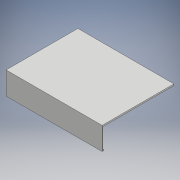
# Autodesk Inventor part: 包包分隔檔板
Saved by Autodesk Inventor 2017 (Build 210142000, 142)
## iProperties
Part Number: 包包分隔檔板
Material: 一般
Document SubType Name: Modeling
Designer: user
Density: 1 g/cm^3
Appearance: 預設
Author: user
Autodesk Inventor part; units mm, degrees
ref_plane "YZ Plane" through (0, 0, 0) normal (1, 0, 0) x (0, 1, 0)
ref_plane "XZ Plane" through (0, 0, 0) normal (0, 1, 0) x (-1, 0, 0)
ref_plane "XY Plane" through (0, 0, 0) normal (0, 0, 1) x (1, 0, 0)
sketch "草圖1" plane through (0, 0, 0) normal (0, 1, 0) x (-1, 0, 0)
  line L0 (0, 0) -> (-254, 0)
  line L1 (-254, 0) -> (-254, 60)
  line L2 (-254, 60) -> (0, 60)
  line L3 (0, 60) -> (0, 0)
  dimension "d0" = 254
  dimension "d1" = 60
  constraints: 8 end point, 2 parallel, 1 horizontal, 1 perpendicular
  measures "d0" distance of L1.end L2.end
  measures "d1" distance of L0.end L1.end
extrude "擠出1" add sketch "草圖1" along normal blind 190
sketch "草圖2" plane through (0, 190, 0) normal (0, 1, 0) x (1, 0, 0)
  line L0 (254, 0) -> (0, 0) projected
  line L1 (0, 0) -> (254, 0)
  line L2 (254, 0) -> (254, -56)
  line L3 (254, -56) -> (0, -56)
  line L4 (0, -56) -> (0, 0)
  dimension "d4" = 254
  dimension "d5" = 56
  constraints: 8 end point, 2 parallel, 1 horizontal, 1 perpendicular
  measures "d4" distance of L2.end L3.end
  measures "d5" distance of L1.end L2.end
extrude "擠出2" cut sketch "草圖2" against normal blind 188
sketch "草圖3" plane through (0, 2, 0) normal (0, 1, 0) x (1, 0, 0)
  line L0 (0, 0) -> (254, 0)
  line L1 (254, 0) -> (254, -2)
  line L2 (254, -2) -> (0, -2)
  line L3 (0, -2) -> (0, 0)
  dimension "d8" = 254
  dimension "d9" = 2
  constraints: 8 end point, 2 parallel, 1 horizontal, 1 perpendicular
  measures "d8" distance of L1.end L2.end
  measures "d9" distance of L0.end L1.end
extrude "擠出3" add sketch "草圖3" along normal blind 2
sketch "草圖4" plane through (0, 2, 2) normal (0, 0, 1) x (1, 0, 0)
  line L0 (0, 2) -> (254, 2) projected
  line L1 (0, 2) -> (254, 2)
  line L2 (254, 2) -> (254, 1.2)
  line L3 (254, 1.2) -> (0, 1.2)
  line L4 (0, 1.2) -> (0, 2)
  point P0 (0, -2)
  dimension "d12" = 254
  dimension "d13" = 0.8
  constraints: 8 end point, 2 parallel, 1 horizontal, 1 perpendicular
  measures "d12" distance of L2.end L3.end
  measures "d13" distance of L1.end L2.end
extrude "擠出4" add sketch "草圖4" along normal blind 0.8
